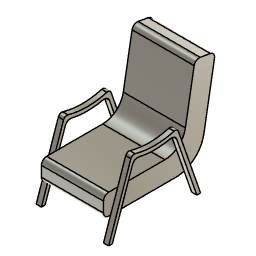
27 (Autodesk Fusion 360 design; units mm, degrees)
Autodesk Fusion 360 part; units mm, degrees
sketch "草图1" plane through (0, 0, 0) normal (1, 0, 0) x (0, 1, 0)
  line L0 (-649.2476, 0) -> (0, 0)
  arc A0 (0, 0) -> (270.8221, 227.2465) centre (0, 275) ccw
  line L1 (270.8221, 227.2465) -> (373.8385, 811.4816)
  arc A1 (373.8385, 811.4816) -> (333.2805, 869.4044) centre (324.5981, 820.164) ccw
  line L2 (333.2805, 869.4044) -> (234.7997, 886.7692)
  arc A2 (234.7997, 886.7692) -> (176.8769, 846.2112) centre (226.1173, 837.5288) ccw
  line L3 (176.8769, 846.2112) -> (92.3655, 366.9231)
  arc A3 (-106.5657, 200) -> (92.3655, 366.9231) centre (-106.5657, 402) ccw
  line L4 (-106.5657, 200) -> (-649.2476, 200)
  arc A4 (-649.2476, 200) -> (-699.2476, 150) centre (-649.2476, 150) ccw
  line L5 (-699.2476, 150) -> (-699.2476, 50)
  arc A5 (-699.2476, 50) -> (-649.2476, 0) centre (-649.2476, 50) ccw
  line L6 (-130, 0) -> (100, 0) construction
  line L7 (373.8385, 811.4816) -> (230.7524, 0) construction
  dimension "d1" = 200
  dimension "d2" = 50
  dimension "d3" = 50
  dimension "d4" = 100
  dimension "d5" = 930
  dimension "d6" = 874
  dimension "d7" = 50
  dimension "d8" = 50
  dimension "d9" = 275
  dimension "d10" = 202
  dimension "d11" = 200
  constraint horizontal L0
  constraint tangent L0 A0
  constraint tangent L1 A1
  constraint tangent L2 A2
  constraint tangent L3 A3
  constraint tangent A3 L4
  constraint tangent L4 A4
  constraint perpendicular L4 L5
  constraint tangent L5 A5
  constraint horizontal L6
  constraint collinear L0 L6
  constraint parallel L0 L4
  constraint parallel L1 L3
  constraint tangent L0 A5
  constraint tangent A4 L5
  constraint coincident L6 L7.end
  constraint tangent A1 L7
  constraint tangent A1 L2
  constraint tangent A2 L3
  constraint tangent A0 L7
  constraint coincident L0.end A0.start
  constraint perpendicular L2 L7
  measures "d1" distance of L0 L4
  measures "d2" radius of A5
  measures "d3" radius of A4
  measures "d4" angle of L3 L4
  measures "d5" distance of L5 L7.end
  measures "d6" distance of L2 L7.end
  measures "d7" radius of A1
  measures "d8" radius of A2
  measures "d9" radius of A0
  measures "d10" radius of A3
  measures "d11" distance of L1 L3
extrude "拉伸1" add sketch "草图1" along normal mid plane 600 makes body 1
sketch "草图2" plane through (300, 0, 0) normal (1, 0, 0) x (0, 1, 0)
  line L0 (-1000, 0) -> (500, 0) construction
  line L1 (-255.2476, 500) -> (-255.2476, -500) construction
  line L2 (-699.2476, 150) -> (-699.2476, 50)
  line L3 (-699.2476, -200) -> (-663.2885, -200)
  line L4 (-663.2885, -200) -> (-468.2546, 366.4195)
  line L5 (-699.2476, -200) -> (-484.7688, 422.8917)
  arc A0 (-443.2224, 444.4975) -> (-484.7688, 422.8917) centre (-452.6211, 411.8224) ccw
  arc A1 (-408.5365, 399.5028) -> (-468.2546, 366.4195) centre (-420.0332, 349.8155) ccw
  arc A2 (-408.5365, 399.5028) -> (-101.9587, 399.5028) centre (-255.2476, 1062) ccw
  arc A3 (-443.2224, 444.4975) -> (-67.2728, 444.4975) centre (-255.2476, 1098) ccw
  arc A4 (-25.7264, 422.8917) -> (-67.2728, 444.4975) centre (-57.8741, 411.8224) ccw
  arc A5 (-42.2406, 366.4195) -> (-101.9587, 399.5028) centre (-90.462, 349.8155) ccw
  line L6 (-42.2406, 366.4195) -> (152.7933, -200)
  line L7 (152.7933, -200) -> (188.7524, -200)
  line L8 (188.7524, -200) -> (-25.7264, 422.8917)
  line L9 (-255.2476, 500) -> (-255.2476, 524.2021) construction
  line L10 (-255.2476, 524.2021) -> (-255.2476, 850) construction
  dimension "d16" = 444
  dimension "d17" = 34
  dimension "d18" = 888
  dimension "d19" = 34
  dimension "d20" = 34
  dimension "d21" = 680
  dimension "d22" = 51
  dimension "d23" = 51
  dimension "d24" = 36
  dimension "d25" = 38
  dimension "d26" = 200
  dimension "d27" = 418
  dimension "d28" = 680
  constraint horizontal L0
  constraint vertical L1
  constraint perpendicular L2 L3
  constraint tangent L5 A0
  constraint tangent L4 A1
  constraint tangent A3 A4
  constraint tangent A2 A5
  constraint horizontal L7
  constraint tangent A5 L6
  constraint tangent A4 L8
  constraint tangent A0 A3
  constraint tangent A1 A2
  constraint collinear L3 L7
  constraint parallel L6 L8
  constraint symmetric L1 L4 L6
  constraint parallel L4 L5
  constraint symmetric L1 L5 L8
  constraint symmetric L1 A0.centre A4.centre
  constraint symmetric L1 A1.centre A5.centre
  constraint coincident L1.start L9.start
  constraint parallel L1 L10
  constraint collinear L1 L9
  measures "d16" distance of L1 L2
  measures "d17" distance of L6 L8
  measures "d18" distance of L3.start L7.end
  measures "d19" radius of A4
  measures "d20" radius of A0
  measures "d21" radius of A3
  measures "d22" radius of A5
  measures "d23" radius of A1
  measures "d24" distance of A2 A3
  measures "d25" angle of L4 L6
  measures "d26" distance of L0 L3.start
  measures "d27" distance of L0 A3
  measures "d28" radius of A2
extrude "拉伸2" add sketch "草图2" along normal blind 50 separate body makes body 2
copy_body "复制和粘贴实体1" bodies 2 makes body 3
move_body "移动1" bodies 3 to x (1, 0, 0) y (0, 1, 0) z (0, 0, 1) at (-650, 0, 0)
combine "合并1" operation add target body 1 tool bodies 3 2
